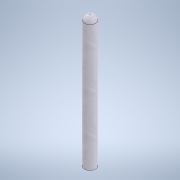
# Autodesk Inventor part: Optical Post
Saved by Autodesk Inventor 2020 (Build 240168000, 168)
## iProperties
Created: 2024-01-30
Part Number: Optical Post
Material: Aluminum 6061, Welded
Document SubType Name: Modeling
Designer: Scott
Density: 2.7 g/cm^3
Appearance: Weld - Aluminum
Mass: 50.6475 g
Surface Area: 61.1933 cm^2
Volume: 18.7583 cm^3
Author: Scott
Autodesk Inventor part; units mm, degrees
ref_plane "YZ Plane" through (0, 0, 0) normal (1, 0, 0) x (0, 1, 0)
ref_plane "XZ Plane" through (0, 0, 0) normal (0, 1, 0) x (-1, 0, 0)
ref_plane "XY Plane" through (0, 0, 0) normal (0, 0, 1) x (1, 0, 0)
sketch "Sketch3" plane through (0, 0, 0) normal (0, 0, 1) x (1, 0, 0)
  line L0 (0, 0) -> (6.35, 0)
  line L1 (0, 0) -> (0, 150)
  line L2 (0, 150) -> (0.35, 150)
  line L3 (6.35, 144) -> (6.35, 0)
  arc A0 (6.35, 144) -> (0.35, 150) centre (0.35, 144) ccw
  dimension "d1" = 6.35
  dimension "d2" = 150
  dimension "d3" = 6
  constraints: 8 end point, 2 perpendicular, 2 point on circle, 2 tangent, 1 centre point, 1 horizontal, 1 vertical
  measures "d1" distance of L0.start L0.end
  measures "d2" distance of L0.start L1.end
  measures "d3" radius of A0
revolve "Revolution1" add sketch "Sketch3" angle 360 about axis through (0, 0, 0) along (0, 1, 0)
body "Solid1"
